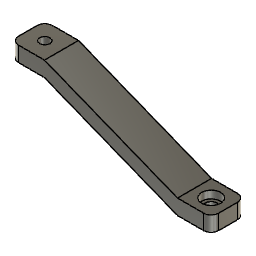
Lenkachse v1 (Autodesk Fusion 360 design; units mm, degrees)
Autodesk Fusion 360 part; units mm, degrees
sketch "Skizze1" plane through (0, 0, 0) normal (0, 0, 1) x (1, 0, 0)
  circle A0 centre (22, 0) radius 1.6
  circle A1 centre (-22, 0) radius 1.35
  line L0 (-25.6, 3.6) -> (25.6, 3.6)
  line L1 (25.6, 3.6) -> (25.6, -3.6)
  line L2 (25.6, -3.6) -> (-25.6, -3.6)
  line L3 (-25.6, -3.6) -> (-25.6, 3.6)
  line L4 (-25.6, 3.6) -> (25.6, -3.6) construction
  line L5 (25.6, 3.6) -> (-25.6, -3.6) construction
  dimension "d5" = 3.2
  dimension "d6" = 2.7
  dimension "d7" = 51.2
  dimension "d8" = 7.2
  constraint horizontal L0
  constraint perpendicular L0 L1
  constraint parallel L0 L2
  constraint parallel L1 L3
  constraint coincident L4 origin
  constraint coincident L5 origin
  measures "d5" diameter of A0
  measures "d6" diameter of A1
  measures "d7" distance of L1.end L2.end
  measures "d8" distance of L0.end L1.end
extrude "Extrusion1" add sketch "Skizze1" along normal blind 10
extrude "Extrusion2" add 1 faces at (-8.575, -2.0516, 10) along direction (0, 0, 1) blind 36
sketch "Skizze2" plane through (0, -3.6, 0) normal (0, -1, 0) x (1, 0, 0)
  line L0 (-25.6, 0) -> (25.6, 0)
  line L1 (25.6, 0) -> (25.6, 46)
  line L2 (25.6, 46) -> (-25.6, 46)
  line L3 (-25.6, 46) -> (-25.6, 0)
  line L4 (25.6, 0) -> (25.6, 28)
  line L5 (-25.6, 46) -> (-17.6, 46)
  line L6 (25.6, 28) -> (17.6, 28)
  line L7 (25.6, 32) -> (17.6, 32)
  line L8 (-25.6, 46) -> (-25.6, 42)
  line L9 (-25.6, 42) -> (-17.6, 42)
  line L10 (25.6, 28) -> (25.6, 32)
  line L11 (17.6, 28) -> (-17.6, 42)
  line L12 (17.6, 32) -> (-17.6, 46)
  dimension "d13" = 28
  dimension "d14" = 8
  dimension "d19" = 8
  dimension "d21" = 8
  dimension "d22" = 4
  dimension "d23" = 8
  constraint coincident L0.end L1.start
  constraint perpendicular L0 L4
  constraint coincident L2.end L3.start
  constraint perpendicular L3 L5
  constraint perpendicular L4 L6
  constraint perpendicular L2 L8
  constraint perpendicular L8 L9
  constraint perpendicular L7 L10
  measures "d13" distance of L0.end L4.end
  measures "d14" distance of L2.end L5.end
  measures "d19" distance of L4.end L6.end
  measures "d21" distance of L7.start L7.end
  measures "d22" distance of L2.end L8.end
  measures "d23" distance of L8.end L9.end
extrude "Extrusion3" cut sketch "Skizze2" against normal blind 9 contours L0 L1 L3 L4 L6 L9 L11 | L1 L2 L7 L12
sketch "Skizze3" plane through (0, 0, 32) normal (0, 0, 1) x (-1, 0, 0)
  line L0 (-25.6, -3.6) -> (-17.6, -3.6)
  line L1 (-17.6, -3.6) -> (-17.6, 3.6)
  line L2 (-17.6, 3.6) -> (-25.6, 3.6)
  line L3 (-25.6, 3.6) -> (-25.6, -3.6)
  circle A0 centre (-22, 0) radius 1.6
  circle A1 centre (-22, 0) radius 2.5
  dimension "d26" = 5
  constraint concentric A0 A1
  measures "d26" diameter of A1
extrude "Extrusion4" cut sketch "Skizze3" against normal blind 2 contours A1
extrude "Extrusion5" add 1 faces at (25.6, 1.2, 29.3333) along direction (1, 0, 0) blind 0.9
extrude "Extrusion6" add 1 faces at (-25.6, -1.2, 43.3333) along direction (-1, 0, 0) blind 0.9
extrude "Extrusion7" add 1 faces at (-5.8667, -3.6, 40) along direction (0, -1, 0) blind 0.9
extrude "Extrusion8" add 1 faces at (-5.8667, 3.6, 40) along direction (0, 1, 0) blind 0.9
chamfer "Fase1" distance 1.15 angle 45 1 edges at (-23.2586, 0.4882, 42)
fillet "Abrundung1" radius 2 4 edges at (-26.5, 4.5, 44) (-26.5, -4.5, 44) (26.5, -4.5, 30) (26.5, 4.5, 30)
move_body "Verschieben1" bodies 1 to x (1, 0, 0) y (0, 1, 0) z (0, 0, 1) at (0, 0, -28)
